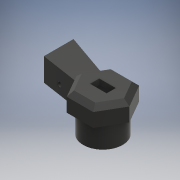
# Autodesk Inventor part: HA09
Saved by Autodesk Inventor 2017 (Build 210142000, 142)
## iProperties
Created: 2019-05-07
Part Number: HA09
Material: ABS Plastic
Document SubType Name: Modeling
Designer: Dell
Density: 1.06 g/cm^3
Appearance: Smooth - Black
Author: Dell
Autodesk Inventor part; units mm, degrees
ref_plane "YZ Plane" through (0, 0, 0) normal (1, 0, 0) x (0, 1, 0)
ref_plane "XZ Plane" through (0, 0, 0) normal (0, 1, 0) x (-1, 0, 0)
ref_plane "XY Plane" through (0, 0, 0) normal (0, 0, 1) x (1, 0, 0)
sketch "Sketch1" plane through (0, 0, 0) normal (0, 0, 1) x (1, 0, 0)
  line L0 (-81.25, 34.5932) -> (-38.1213, 34.5932)
  line L1 (-81.25, 15.0318) -> (-81.25, 34.5932)
  line L2 (-81.25, 15.0318) -> (-81.25, 15.0318)
  line L3 (-21.7063, 5.9235) -> (-81.25, 15.0318)
  arc A0 (-2.8348, 22.3207) -> (-21.7063, 5.9235) centre (0, 0) ccw
  line L4 (-38.1213, 34.5932) -> (-2.8348, 22.3207)
  line L5 (-81.25, 49.5932) -> (-38.1213, 34.5932)
  line L6 (-81.25, 49.5932) -> (-81.25, 49.5932)
  line L7 (-81.25, 49.5932) -> (-81.25, 34.5932)
  line L8 (-81.25, 34.5932) -> (-38.1213, 34.5932)
  circle A1 centre (0, 0) radius 22.5
  line L9 (-81.25, -28.9198) -> (-81.25, 67.2697)
  line L10 (-81.25, 49.5932) -> (-81.25, 15.0318)
  dimension "d0" = 81.25
  constraints: 22 end point, 3 point on line, 2 point on circle, 2 vertical, 1 centre point, 1 coincident, 3 other
  measures "d0" distance from line of point (0, 0) L9
extrude "Extrusion1" add sketch "Sketch1" along normal blind 25
sketch "Sketch5" plane through (0, 0, 0) normal (0, 0, -1) x (-1, 0, 0)
  line L0 (81.25, 49.5932) -> (81.25, 15.0318) projected
  line L1 (2.8348, 22.3207) -> (81.25, 49.5932) projected
  arc A0 (2.8348, 22.3207) -> (21.7063, 5.9235) centre (0, 0) ccw projected
  line L2 (81.25, 15.0318) -> (21.7063, 5.9235) projected
  arc A1 (3.295, 17.187) -> (14.4499, 9.8717) centre (0, 0) ccw
  line L3 (3.295, 17.187) -> (76.25, 42.5605)
  line L4 (76.25, 42.5605) -> (76.25, 19.3251)
  line L5 (76.25, 19.3251) -> (14.4499, 9.8717)
  dimension "d14" = 5
  constraints: 6 end point, 2 point on circle, 1 centre point, 3 other
  measures "d14" distance between parallel lines of L2 L5
extrude "Extrusion5" cut sketch "Sketch5" against normal blind 22 contours L3 L4 L5 A1
sketch "Sketch6" plane through (0, 0, 0) normal (0, 0, -1) x (-1, 0, 0)
  arc A0 (2.8348, 22.3207) -> (21.7063, 5.9235) centre (0, 0) ccw projected
  line L0 (76.25, 19.3251) -> (14.4499, 9.8717) projected
  arc A1 (3.295, 17.187) -> (14.4499, 9.8717) centre (0, 0) ccw projected
  line L1 (3.295, 17.187) -> (76.25, 42.5605) projected
  line L2 (76.25, 42.5605) -> (76.25, 19.3251) projected
  line L3 (81.25, 49.5932) -> (81.25, 15.0318) projected
  line L4 (2.8348, 22.3207) -> (81.25, 49.5932) projected
  arc A2 (2.8348, 22.3207) -> (21.7063, 5.9235) centre (0, 0) ccw projected
  line L5 (81.25, 15.0318) -> (21.7063, 5.9235) projected
  line L6 (80.25, 48.1867) -> (80.25, 15.8905)
  line L7 (80.25, 15.8905) -> (20.4169, 6.7379)
  arc A3 (2.939, 21.2982) -> (20.4169, 6.7379) centre (0, 0) ccw
  line L8 (2.939, 21.2982) -> (80.25, 48.1867)
  dimension "d17" = 1
  constraints: 6 end point, 2 point on circle, 1 centre point, 3 other
  measures "d17" distance between parallel lines of L4 L8
extrude "Extrusion6" cut sketch "Sketch6" against normal through all contours L4 L3 L5 A0
sketch "Sketch7" plane through (0, 0, 25) normal (0, 0, 1) x (1, 0, 0)
  line L0 (9, -5) -> (-9, -5)
  line L1 (-9, -5) -> (-9, 5)
  line L2 (-9, 5) -> (9, 5)
  line L3 (9, 5) -> (9, -5)
  point P0 (0, 0)
  point P1 (0, -5)
  point P2 (-9, 0)
  dimension "d20" = 18
  dimension "d21" = 10
  constraints: 8 end point, 2 midpoint, 2 parallel, 1 horizontal, 1 horizontal alignment, 1 perpendicular, 1 vertical alignment
  measures "d20" distance of L1.end L2.end
  measures "d21" distance of L0.end L1.end
extrude "Extrusion7" cut sketch "Sketch7" against normal through all
sketch "Sketch8" plane through (-9, -5, 25) normal (0, 1, 0) x (1, 0, 0)
  circle A0 centre (-51, 15) radius 2.5
  line L0 (-12.5, 0) -> (30.5, 0) projected
  point P0 (9, 25)
  point P1 (-11.4169, 0)
  point P2 (6.061, 0)
  dimension "d24" = 5
  dimension "d25" = 60
  dimension "d26" = 15
  constraints: 1 centre point
  measures "d24" diameter of A0
  measures "d25" horizontal distance of A0.centre point (9, 25)
  measures "d26" distance from line of A0.centre L0
extrude "Extrusion8" cut sketch "Sketch8" along normal through all
sketch "Sketch9" plane through (0, 0, 25) normal (0, 0, 1) x (1, 0, 0)
  arc A0 (-20.4169, 6.7379) -> (-2.939, 21.2982) centre (0, 0) ccw projected
  circle A1 centre (0, 0) radius 21.5
  line L0 (28.8675, 0) -> (14.4338, -25)
  line L1 (14.4338, -25) -> (-14.4338, -25)
  line L2 (-14.4338, -25) -> (-28.8675, 0)
  line L3 (-28.8675, 0) -> (-14.4338, 25)
  line L4 (-14.4338, 25) -> (14.4338, 25)
  line L5 (14.4338, 25) -> (28.8675, 0)
  line L6 (9, 5) -> (9, -5) projected
  line L7 (-9, 5) -> (9, 5) projected
  line L8 (-9, -5) -> (-9, 5) projected
  line L9 (9, -5) -> (-9, -5) projected
  dimension "d31" = 50
  constraints: 12 end point, 2 coincident, 1 horizontal alignment, 16 other
  measures "d31" distance between parallel lines of L1 L4
extrude "Extrusion9" add sketch "Sketch9" along normal blind 20 contours A1 A0 | L0 L1 L2 L3 L4 L5
sketch "Sketch10" plane through (-76.25, 19.3251, 0) normal (1, 0, 0) x (0, 0, -1)
  line L0 (0, 23.2353) -> (0, 0) projected
  line L1 (0, 23.2353) -> (-22, 23.2353) projected
  line L2 (-22, 23.2353) -> (-22, 0) projected
  line L3 (0, 0) -> (-22, 0) projected
  line L4 (0, -3.4347) -> (0, 28.8615) projected
  line L5 (0, 16.6177) -> (-10, 16.6177)
  line L6 (-10, 16.6177) -> (-10, 6.6177)
  line L7 (-10, 6.6177) -> (0, 6.6177)
  line L8 (0, 6.6177) -> (0, 16.6177)
  point P0 (0, -19.3251)
  point P1 (0, 11.6177)
  dimension "d32" = 10
  dimension "d33" = 10
  constraints: 8 end point, 2 midpoint, 2 parallel, 1 horizontal, 1 perpendicular, 1 point on line
  measures "d32" distance of L5.start L5.end
  measures "d33" distance between parallel lines of L7 L5
extrude "Extrusion10" cut sketch "Sketch10" against normal through all contours L0 L7 L6 L5
chamfer "Chamfer1" distance 2 angle 45 4 edges at (-78.25, 35.9428, 0) (-78.25, 25.9428, 0) (-78.25, 35.9428, 10) (-78.25, 25.9428, 10)
sketch "Sketch11" plane through (-80.25, 48.1867, 25) normal (0.3284957, 0.9445055, 0) x (0.9445055, -0.3284957, 0)
  line L0 (70.1284, 25) -> (10.6092, 25) projected
  line L1 (70.1284, 25) -> (0, 17)
  line L2 (0, 25) -> (0, 0) projected
  line L3 (0, 17) -> (0, 25)
  line L4 (0, 25) -> (70.1284, 25)
  point P0 (91.6257, 25)
  dimension "d39" = 8
  constraints: 6 end point, 1 collinear, 1 perpendicular, 1 point on line
  measures "d39" distance from line of L1.end L4
extrude "Extrusion11" cut sketch "Sketch11" against normal blind 15
sketch "Sketch12" plane through (0, 0, 22) normal (0, 0, -1) x (-1, 0, 0)
  arc A0 (3.295, 17.187) -> (14.4499, 9.8717) centre (0, 0) ccw projected
  circle A1 centre (0, 0) radius 17.5
  constraints: 1 coincident, 3 other
extrude "Extrusion12" cut sketch "Sketch12" against normal blind 15
chamfer "Chamfer2" distance 5 angle 45 6 edges at (0, -25, 45) (21.6506, -12.5, 45) (-21.6506, -12.5, 45) (-21.6506, 12.5, 45) (0, 25, 45) (21.6506, 12.5, 45)
chamfer "Chamfer3" distance 2 angle 45 4 edges at (0, 5, 37) (-9, 0, 37) (0, -5, 37) (9, 0, 37)
fillet "Fillet1" radius 4 1 edges at (-47.1317, 36.6682, 4)
body "Solid1"
